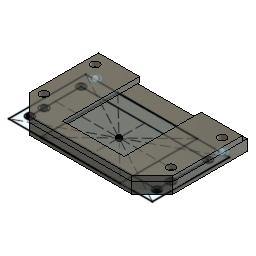
Duale3Pro breakboard fixing v4 (Autodesk Fusion 360 design; units mm, degrees)
Autodesk Fusion 360 part; units mm, degrees
note: some values were not read from the file. Set by a fixed rule: which sketch regions a step uses.
sketch "Breakboard Backplate" plane through (0, 0, 0) normal (0, 1, 0) x (1, 0, 0)
  line L0 (0, 0) -> (49.5, 0)
  line L1 (49.5, 0) -> (49.5, 20)
  line L2 (49.5, 20) -> (0, 20)
  line L3 (0, 20) -> (0, 0)
  circle A0 centre (0, 0) radius 1.5
  line L4 (0, 10) -> (49.5, 10) construction
  line L5 (24.75, 20) -> (24.75, 0) construction
  circle A1 centre (0, 20) radius 1.5
  circle A2 centre (49.5, 20) radius 1.5
  circle A3 centre (49.5, 0) radius 1.5
  line L6 (52.75, 25) -> (-3.25, 25)
  line L7 (-3.25, 25) -> (-3.25, -5)
  line L8 (-3.25, -5) -> (52.75, -5)
  line L9 (52.75, -5) -> (52.75, 25)
  line L10 (52.75, 25) -> (-3.25, -5) construction
  line L11 (-3.25, 25) -> (52.75, -5) construction
  line L12 (40.25, 25) -> (9.25, 25)
  line L13 (9.25, 25) -> (9.25, -5)
  line L14 (9.25, -5) -> (40.25, -5)
  line L15 (40.25, -5) -> (40.25, 25)
  line L16 (40.25, 25) -> (9.25, -5) construction
  line L17 (9.25, 25) -> (40.25, -5) construction
  circle A4 centre (0, 5.5) radius 1.6
  circle A5 centre (49.5, 5.5) radius 1.6
  circle A6 centre (0, 25.5) radius 1.6
  circle A7 centre (49.5, 25.5) radius 1.6
  point P0 (24.75, 10)
  point P1 (24.75, 10)
  dimension "d1" = 49.5
  dimension "d2" = 20
  dimension "d3" = 3
  dimension "d6" = 3.25
  dimension "d7" = 5
  dimension "d8" = 31
  dimension "d31" = 3.2
  dimension "d32" = 5.5
  constraint horizontal L0
  constraint vertical L1
  constraint horizontal L2
  constraint vertical L3
  constraint coincident L0.start L3.end
  constraint midpoint L3 L4.start
  constraint midpoint L1 L4.end
  constraint midpoint L2 L5.start
  constraint midpoint L0 L5.end
  constraint symmetric A0 L4 A1
  constraint symmetric A0 L5 A3
  constraint symmetric L5 A1 A2
  constraint perpendicular L6 L7
  constraint parallel L6 L8
  constraint parallel L7 L9
  constraint horizontal L6
  constraint coincident L10 P1
  constraint coincident L11 P1
  constraint midpoint L4 P1
  constraint perpendicular L12 L13
  constraint parallel L12 L14
  constraint parallel L13 L15
  constraint horizontal L12
  constraint coincident L6 L12.start
  constraint coincident L16 P1
  constraint coincident L17 P1
  constraint coincident P1 P0
  constraint coincident L3 A4.centre
  constraint symmetric L5 A4 A5
  constraint equal A4 A6
  constraint equal A5 A7
  measures "d1" distance of L0.start L0.end
  measures "d2" distance of L0.start L2.end
  measures "d3" diameter of A0
  measures "d6" distance of L1 L9
  measures "d7" distance of L0 L8
  measures "d8" distance of L13.end L14.end
  measures "d31" diameter of A4
  measures "d32" distance of L0.start A4.centre
sketch "Breakboard frontplate" plane through (0, 0, 0) normal (0, 1, 0) x (1, 0, 0)
  line L0 (-3.25, -5) -> (52.75, -5)
  line L1 (52.75, -5) -> (52.75, 25)
  line L2 (52.75, 25) -> (-3.25, 25)
  line L3 (-3.25, 25) -> (-3.25, -5)
  line L4 (-3.25, -5) -> (12.75, -5)
  line L5 (12.75, -5) -> (12.75, 25)
  line L6 (12.75, 25) -> (-3.25, 25)
  line L7 (-3.25, 25) -> (-3.25, -5)
  line L8 (24.75, 10) -> (24.75, 25) construction
  line L9 (24.75, 20) -> (24.75, 0) construction
  line L10 (36.75, -5) -> (36.75, 25)
  line L11 (0, 0) -> (49.5, 0) construction
  line L12 (49.5, 0) -> (49.5, 20) construction
  line L13 (49.5, 20) -> (0, 20) construction
  line L14 (0, 20) -> (0, 0) construction
  line L15 (0, 0) -> (49.5, 20) construction
  line L16 (49.5, 0) -> (0, 20) construction
  line L17 (24.75, 10) -> (-3.25, 10) construction
  circle A0 centre (0, 0) radius 1.5
  circle A1 centre (0, 20) radius 1.5
  circle A2 centre (49.5, 20) radius 1.5
  circle A3 centre (49.5, 0) radius 1.5
  line L18 (12.75, 0) -> (36.75, 0)
  point P0 (-3.25, -5)
  point P1 (52.75, 25)
  point P2 (24.75, 10)
  point P3 (24.75, 10)
  dimension "d9" = 16
  dimension "d10" = 30
  dimension "d11" = 3
  constraint horizontal L0
  constraint vertical L1
  constraint horizontal L2
  constraint vertical L3
  constraint coincident P1 L1.end
  constraint coincident P0 L0.start
  constraint horizontal L4
  constraint vertical L5
  constraint horizontal L6
  constraint vertical L7
  constraint coincident P3 P2
  constraint midpoint L2 L8.end
  constraint symmetric L4.end L9 L10.start
  constraint symmetric L5.end L9 L10.end
  constraint perpendicular L11 L12
  constraint parallel L11 L13
  constraint parallel L12 L14
  constraint horizontal L11
  constraint coincident L11.start L14.end
  constraint coincident L15 P3
  constraint coincident L16 P3
  constraint midpoint L3 L17.end
  constraint symmetric L17 A0 A1
  constraint symmetric L8 A0 A3
  constraint symmetric L8 A1 A2
  constraint coincident L11 L18.start
  constraint coincident L5 L18.start
  constraint coincident L11 L18.end
  constraint coincident L10 L18.end
  measures "d9" distance of P0 L4.end
  measures "d10" distance of P0 L2.end
  measures "d11" diameter of A0
sketch "Breakboard strap" plane through (0, 0, 0) normal (0, 1, 0) x (1, 0, 0)
  line L0 (12.75, 0) -> (36.75, 0)
  line L1 (36.75, 0) -> (36.75, 40)
  line L2 (36.75, 40) -> (12.75, 40)
  line L3 (12.75, 40) -> (12.75, 0)
  circle A0 centre (0, 0) radius 1.375
  line L4 (0, 20) -> (0, 0) construction
  line L5 (0, 10) -> (24.75, 10) construction
  line L6 (24.75, 10) -> (24.75, 40) construction
  line L7 (24.75, 10) -> (-3.25, 10) construction
  circle A1 centre (0, 20) radius 1.375
  circle A2 centre (49.5, 20) radius 1.375
  circle A3 centre (49.5, 0) radius 1.375
  circle A4 centre (0, 0) radius 3.375
  circle A5 centre (0, 20) radius 3.375
  circle A6 centre (49.5, 20) radius 3.375
  circle A7 centre (49.5, 0) radius 3.375
  line L8 (24.75, 40) -> (24.75, 0) construction
  line L9 (22.25, 40) -> (22.25, 0)
  line L10 (27.25, 40) -> (27.25, 0)
  line L11 (12.75, 40) -> (3.5368, 19.63)
  line L12 (0, 0) -> (0, -3.375) construction
  line L13 (0, -3.375) -> (49.5, -3.375)
  line L14 (3.0932, 17.4889) -> (3.2956, 4.9453)
  line L15 (36.75, 40) -> (46.4249, 18.6092)
  line L16 (46.4249, 18.6092) -> (46.2044, 4.9453)
  line L17 (24.75, 45) -> (10.1841, 45)
  line L18 (6.5395, 42.6484) -> (-3.0751, 21.3908)
  line L19 (0, 20) -> (-0.5, 20) construction
  line L20 (-0.5, 20) -> (-3.375, 20) construction
  line L21 (-3.375, 20) -> (-3.375, 0)
  line L22 (24.75, 40) -> (24.75, 45) construction
  line L23 (42.9605, 42.6484) -> (52.5751, 21.3908)
  line L24 (24.75, 45) -> (39.3159, 45)
  line L25 (52.875, 20) -> (52.875, 0)
  line L26 (12.75, 0) -> (8.2659, 0.026)
  line L27 (36.75, 0) -> (41.2341, 0.026)
  arc A8 (3.2956, 4.9453) -> (8.2659, 0.026) centre (8.295, 5.026) ccw
  arc A9 (3.5368, 19.63) -> (3.0932, 17.4889) centre (8.0925, 17.5695) ccw
  arc A10 (3.5368, 19.63) -> (3.0932, 17.4889) centre (8.0925, 17.5695) ccw
  arc A11 (41.2341, 0.026) -> (46.2044, 4.9453) centre (41.205, 5.026) ccw
  arc A12 (10.1841, 45) -> (6.5395, 42.6484) centre (10.1841, 41) ccw
  arc A13 (42.9605, 42.6484) -> (39.3159, 45) centre (39.3159, 41) ccw
  point P0 (12.75, 0)
  point P1 (24.75, 10)
  point P2 (24.75, 0)
  dimension "d12" = 24
  dimension "d13" = 40
  dimension "d14" = 2.75
  dimension "d15" = 2
  dimension "d16" = 2.5
  dimension "d19" = 5
  dimension "d20" = 4
  constraint horizontal L0
  constraint vertical L1
  constraint horizontal L2
  constraint vertical L3
  constraint coincident P0 L0.start
  constraint coincident A0.centre L4.end
  constraint midpoint L4 L5.start
  constraint coincident P1 L5.end
  constraint midpoint L2 L6.end
  constraint symmetric A0 L7 A1
  constraint symmetric A0 L6 A3
  constraint symmetric L6 A1 A2
  constraint symmetric L5 A4 A5
  constraint symmetric L6 A4 A7
  constraint symmetric L6 A5 A6
  constraint coincident P2 L8.end
  constraint symmetric L8 L9.start L10.start
  constraint symmetric L8 L9.end L10.end
  constraint tangent A5 L11
  constraint coincident A4 L12.end
  constraint parallel L4 L12
  constraint coincident A7 L13.end
  constraint tangent A7 L13
  constraint perpendicular L12 L13
  constraint tangent A4 L14
  constraint symmetric L2.end L8 L1.end
  constraint parallel L11 L18
  constraint coincident L4.start A1.centre
  constraint perpendicular L4 L19
  constraint coincident A5 L20.end
  constraint perpendicular L4 L20
  constraint coincident A4 L21.end
  constraint tangent A4 L21
  constraint perpendicular L17 L22
  constraint parallel L2 L17
  constraint symmetric L8 L18.end L23.end
  constraint symmetric L8 L20.end L25.start
  constraint symmetric L8 L21.end L25.end
  constraint symmetric L8 L17.start L22.end
  constraint symmetric P0 L8 L0.end
  constraint tangent L14 A8
  constraint tangent L26 A8
  constraint tangent L14 A9
  constraint tangent L11 A9
  constraint equal A8 A9
  constraint coincident L11 A9.start
  constraint coincident L14 A9.end
  constraint tangent L11 A10
  constraint tangent L27 A11
  constraint tangent L16 A11
  constraint equal A8 A11
  constraint tangent L18 A12
  constraint tangent L17 A12
  constraint tangent L24 A13
  constraint tangent L23 A13
  constraint equal A12 A13
  measures "d12" distance of P0 L0.end
  measures "d13" distance of P0 L2.end
  measures "d14" diameter of A0
  measures "d19" radius of A8
  measures "d20" radius of A12
extrude "Extrude1" add sketch "Breakboard Backplate" against normal blind 1.5 contours L0 L3 A0 | L0 L3 A0 | L0 L2 L3 A0 A1 L13 A4 | L0 L2 L3 A0 A1 L6 L7 L8 L13 A4 A6 | L0 L2 L13 L15 | L0 L8 L13 L14 L15 | L3 A4 | L3 A4 | L0 L1 L2 A2 A3 L15 A5 | L0 L1 L2 A2 A3 L6 L8 L9 L15 A5 A7 | L2 L6 L12 L13 L15 | L0 L1 A3 | L0 L1 A3 | L2 L3 A1 | L2 L3 A1 | L1 L2 A2 | L1 L2 A2 | L6 A6 | L1 A5 | L1 A5 | L6 A7 picked at (0.0393, 24.6348) picked at (49.1434, 24.7266) makes body 1
extrude "Extrude2" add sketch "Breakboard Backplate" along normal blind 2.75 contours L0 L3 A0 | L0 L3 A0 | L0 L2 L3 A0 A1 L13 A4 | L0 L2 L3 A0 A1 L6 L7 L8 L13 A4 A6 | L0 L8 L13 L14 L15 | L3 A4 | L3 A4 | L0 L1 L2 A2 A3 L15 A5 | L0 L1 L2 A2 A3 L6 L8 L9 L15 A5 A7 | L0 L1 A3 | L0 L1 A3 | L2 L3 A1 | L2 L3 A1 | L1 L2 A2 | L1 L2 A2 | L6 A6 | L1 A5 | L1 A5 | L6 A7 picked at (0.0393, 24.6348) picked at (49.1434, 24.7266) bodies 1
extrude "Extrude3" add 1 faces at (48.5833, 0.4167, -25) along direction (0, 0, -1) blind 7 on bodies 1 bodies 1
extrude "Extrude4" add sketch "Breakboard frontplate" sketch "Breakboard Backplate" along normal blind 2 separate body contours L0 L2 L3 L4 L5 L6 L7 | L0 L5 L10 L18 | L0 L1 L2 L10 | A0 | A2 | A3 of sketch 2 contours L0 L3 A0 | L0 L1 A3 | L2 L3 A1 | L2 L3 A1 picked at (0.9946, -0.0734) picked at (48.5056, -0.0745) makes body 2
move_body "Move1" bodies 2 to x (1, 0, 0) y (0, 1, 0) z (0, 0, 1) at (0, 2.75, 0)
extrude "Extrude5" add sketch "Breakboard strap" along normal blind 3 separate body contours A4 A5 A6 A7 L13 L17 L18 L21 L23 L24 L25 A12 A13 | A6 | L0 L2 L9 L10 | A7 | A4 | A5 makes body 3
move_body "Move2" bodies 3 to x (1, 0, 0) y (0, 1, 0) z (0, 0, 1) at (0, 5.25, 0)
move_face "OffsetFaces1" offset 5 2 faces at (47.4167, 4.0833, -25) (7.4167, 4.0833, -25) on bodies 2
extrude "Extrude6" cut sketch "Breakboard Backplate" against normal blind 4 contours L3 A4 | L3 A4 | L6 A6 | L6 A6 | L1 A5 | L1 A5 | L6 A7 | L6 A7 bodies 1
extrude "Extrude7" cut sketch "Breakboard Backplate" along normal blind 10 contours L3 A4 | L3 A4 | L6 A6 | L6 A6 | L1 A5 | L1 A5 | L6 A7 | L6 A7 bodies 1 2
chamfer "Chamfer1" distance 8 angle 45 2 edges at (-3.25, 3.75, 5) (52.75, 3.75, 5) on bodies 2
chamfer "Chamfer2" distance 8 angle 45 2 edges at (-3.25, 0.625, 5) (52.75, 0.625, 5) on bodies 1
hidden bodies 3
named bodies: "Breakboard backplate", "Breakboard frontplate", "Breakboard strap"
